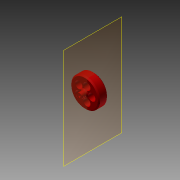
# Autodesk Inventor part: llantasumo
Saved by Autodesk Inventor 2015 (Build 190159000, 159)
## iProperties
Created: 2015-02-17
Part Number: llantasumo
Material: Plástico ABS
Document SubType Name: Modeling
Designer: Víctor
Mass: 45.4313 g
Surface Area: 177.665 cm^2
Volume: 127.161 cm^3
Density: 1.06 g/cm^3
Appearance: Suave - Blanco
Author: Víctor
Autodesk Inventor part; units mm, degrees
ref_plane "XZ Plane" through (0, 0, 0) normal (0, 1, 0) x (-1, 0, 0)
ref_plane "XY Plane" through (0, 0, 0) normal (0, 0, 1) x (1, 0, 0)
sketch "Boceto1" plane through (0, 0, 0) normal (0, 0, 1) x (1, 0, 0)
  circle A0 centre (0, 0) radius 3
  circle A1 centre (0, 0) radius 7.5
  circle A2 centre (0, 0) radius 127
  circle A3 centre (0, 0) radius 31.75 construction
  dimension "d0" = 6
  dimension "d1" = 15
  dimension "d2" = 254
  dimension "d3" = 63.5
  constraints: 4 centre point, 4 coincident
  measures "d0" diameter of A0
  measures "d1" diameter of A1
  measures "d2" diameter of A2
  measures "d3" diameter of A3
extrude "Extrusión1" add sketch "Boceto1" along normal blind 40 contours A1
sketch "Boceto2" plane through (0, 0, 0) normal (0, 0, -1) x (-1, 0, 0)
  circle A0 centre (0, 0) radius 40
  dimension "d6" = 80
  constraints: 1 centre point, 1 coincident
  measures "d6" diameter of A0
extrude "Extrusión2" add sketch "Boceto2" against normal blind 25
ref_plane "Plano de trabajo1" through (7.5, 0, 0) normal (1, 0, 0) x (0, 1, 0)
sketch "Boceto5" plane through (7.5, 0, 0) normal (1, 0, 0) x (0, 1, 0)
  line L0 (7.5, 40) -> (-7.5, 40) projected
  line L1 (0, 40) -> (0, 35)
  point P0 (0, 0)
  dimension "d31" = 5
  constraints: 2 end point, 1 coincident, 1 midpoint, 1 vertical
  measures "d31" distance of L1.start L1.end
sketch "Boceto6" plane through (0, 0, 0) normal (0, 0, -1) x (-1, 0, 0)
  point P0 (0, 0)
  point P1 (0, 0)
  constraints: 1 coincident
hole "Agujero2" at (0, 0, 0) direction (0, 0, 1) diameter 6 end through all
hole "Agujero3" at (7.5, 0, 35) direction (-1, 0, 0) diameter 2.4892 depth 8 tip angle 118
sketch "Boceto7" plane through (0, 0, 0) normal (0, 0, -1) x (-1, 0, 0)
  line L0 (-40, 0) -> (-30, 0)
  line L1 (10, 0) -> (-10, 0)
  line L2 (-30, 0) -> (-10, 0)
  line L3 (-10, 0) -> (-20, 0)
  circle A0 centre (-20, 0) radius 10
  point P0 (0, 0)
  point P1 (-6.1803, -19.0211)
  point P2 (16.1803, -11.7557)
  point P3 (16.1803, 11.7557)
  point P4 (-6.1803, 19.0211)
  dimension "d48" = 10
  dimension "d49" = 40
  dimension "d50" = 20
  dimension "d51" = 20
  dimension "d52" = 10
  dimension "d55" = 360
  constraints: 8 end point, 2 coincident, 1 collinear, 1 horizontal alignment, 1 midpoint, 8 other
  measures "d48" distance of L0.start L0.end
  measures "d49" distance of L0.end L1.start
  measures "d50" distance of L1.start L1.end
  measures "d51" distance of L0.end L1.end
  measures "d52" distance of L1.end L3.end
hole "Agujero4" at (-16.1803, -11.7557, 0) at (6.1803, -19.0211, 0) at (20, 0, 0) at (6.1803, 19.0211, 0) at (-16.1803, 11.7557, 0) direction (0, 0, 1) diameter 20 end through all
chamfer "Chaflán1" distance 3.175 angle 45 1 edges at (-7.5, 0, 25)
chamfer "Chaflán2" distance 3.175 angle 45 2 edges at (40, 0, 25) (40, 0, 0)
